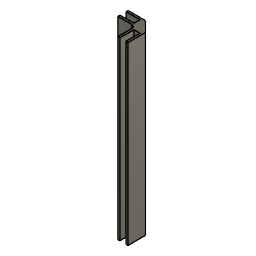
connettore_90_gradi (Autodesk Fusion 360 design; units mm, degrees)
Autodesk Fusion 360 part; units mm, degrees
sketch "Schizzo1" plane through (0, 0, 0) normal (0, 0, 1) x (1, 0, 0)
  line L0 (0, 0) -> (-25, 0)
  line L1 (-25, 0) -> (-25, 3)
  line L2 (-25, 3) -> (-5, 3)
  line L3 (-5, 3) -> (-5, 11.5)
  line L4 (-5, 11.5) -> (-25, 11.5)
  line L5 (-25, 11.5) -> (-25, 14.5)
  line L6 (-25, 14.5) -> (0, 14.5)
  line L7 (0, 14.5) -> (0, 0)
  line L8 (14.5, 0) -> (14.5, -25)
  line L9 (11.5, -5) -> (3, -5)
  line L10 (0, 0) -> (14.5, 0)
  line L11 (0, -25) -> (0, 0)
  line L12 (3, -5) -> (3, -25)
  line L13 (14.5, -25) -> (11.5, -25)
  line L14 (3, -25) -> (0, -25)
  line L15 (11.5, -25) -> (11.5, -5)
  line L16 (0, 14.5) -> (14.5, 0)
  point P0 (14.5, 0)
  dimension "d2" = 8.5
  dimension "d3" = 3
  dimension "d4" = 3
  dimension "d5" = 25
  dimension "d6" = 25
  dimension "d7" = 20
  dimension "d8" = 8.5
  dimension "d9" = 3
  dimension "d10" = 3
  dimension "d11" = 25
  dimension "d12" = 25
  dimension "d13" = 20
  dimension "d16" = 90
  constraint coincident L0.start L7.end
  constraint horizontal L0
  constraint perpendicular L0 L1
  constraint perpendicular L1 L2
  constraint perpendicular L2 L3
  constraint perpendicular L3 L4
  constraint perpendicular L4 L5
  constraint perpendicular L5 L6
  constraint perpendicular L0 L7
  constraint coincident P0 L8.start
  constraint perpendicular L8 L13
  constraint perpendicular L13 L15
  constraint perpendicular L9 L15
  constraint perpendicular L9 L12
  constraint perpendicular L12 L14
  constraint perpendicular L11 L14
  constraint perpendicular L8 L10
  measures "d2" distance of L2.end L3.end
  measures "d3" distance of L4.end L5.end
  measures "d4" distance of L0.end L1.end
  measures "d5" distance of L0.start L0.end
  measures "d6" distance of L5.end L6.end
  measures "d7" distance of L1.end L2.end
  measures "d8" distance of L9.start L9.end
  measures "d9" distance of L12.end L11.start
  measures "d10" distance of L13.end L8.end
  measures "d11" distance of P0 L8.end
  measures "d12" distance of L11.start L0.start
  measures "d13" distance of L13.end L9.start
  measures "d16" angle of L7 L10
extrude "Estrusione1" add sketch "Schizzo1" along normal blind 250
fillet "Raccordo1" radius 5 1 edges at (0, 0, 125)
